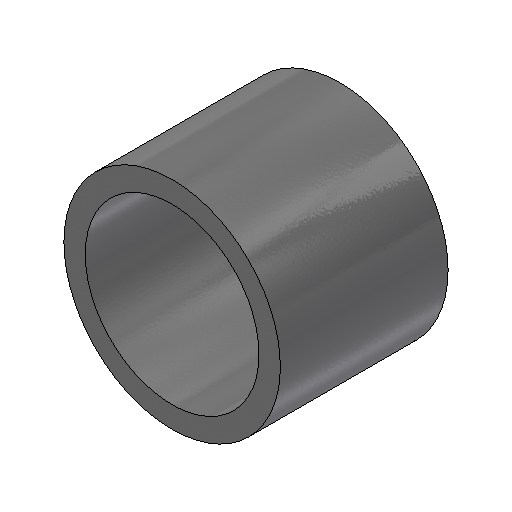
# Autodesk Inventor part: TL20240901-10320CV-010
Saved by Autodesk Inventor 2022.5 (Build 265521000, 521)
## iProperties
Category: FOLLOWER UNIT ASSY
Manager: 호상태
Company: 현대 트랜시스
Created: 2023-01-26
Part Number: TL20240901-10320CV-010
Checked By: 김형민
Engr Approved By: 김형민
User Status: 2 x6
Material: S45C
Description: 0
Document SubType Name: Modeling
Mfg Approved By: 호상태
Designer: 박성규
Stock Number: 010
Density: 7.87 g/cm^3
Appearance: Plating Zinc White
Project: MEa-PJT 2LINE
DETAIL: Coveryor Assembly
M/C TITLE: MEa/NEa차종 시트조립라인
SPECIFICATION: TL20221201-000000CV-035
DocNumber: 221118_Standard_v1
Folder: .\
VDS_Category: 엔지니어링
Detail Description: Processed products
Title: COLLAR
Subject: MEa차종 시트조립2라인
Author: 박성규
Revision Number: A
Autodesk Inventor part; units mm, degrees
ref_plane "YZ Plane" through (0, 0, 0) normal (1, 0, 0) x (0, 1, 0)
ref_plane "XZ Plane" through (0, 0, 0) normal (0, 1, 0) x (-1, 0, 0)
ref_plane "XY Plane" through (0, 0, 0) normal (0, 0, 1) x (1, 0, 0)
sketch "스케치8" plane through (0, 0, 0) normal (0, 0, 1) x (1, 0, 0)
  circle A0 centre (0, 0) radius 16.05
  circle A1 centre (0, 0) radius 20
  dimension "d38" = 40
  dimension "d39" = 32.1
  constraints: 2 centre point, 2 coincident
  measures "d38" diameter of A1
  measures "d39" diameter of A0
extrude "돌출3" add sketch "스케치8" along normal blind 31
